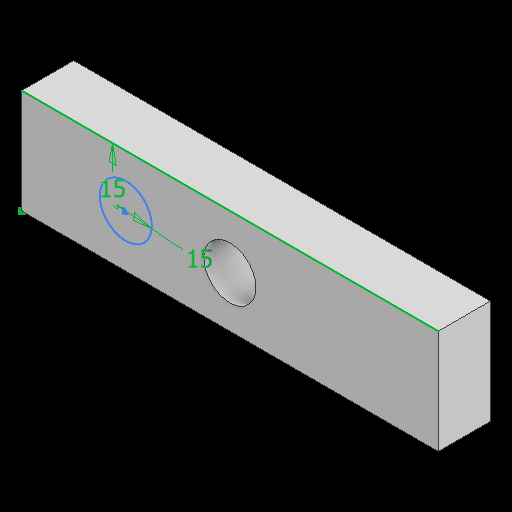
# Autodesk Inventor part: lever1.2
Saved by Autodesk Inventor 2025.1 (Build 291241000, 241)
## iProperties
Created: 2024-08-22
Part Number: lever1.2
Material: 일반
Document SubType Name: Modeling
Designer: ojs08
Density: 1 g/cm^3
Appearance: 기본값
Author: ojs08
Autodesk Inventor part; units mm, degrees
ref_plane "YZ Plane" through (0, 0, 0) normal (1, 0, 0) x (0, 1, 0)
ref_plane "XZ Plane" through (0, 0, 0) normal (0, 1, 0) x (-1, 0, 0)
ref_plane "XY Plane" through (0, 0, 0) normal (0, 0, 1) x (1, 0, 0)
sketch "스케치1" plane through (0, 0, 0) normal (0, 0, 1) x (1, 0, 0)
  line L0 (0, 30) -> (120, 30)
  line L1 (120, 30) -> (120, 0)
  line L2 (120, 0) -> (0, 0)
  line L3 (0, 0) -> (0, 30)
  dimension "d0" = 120
  dimension "d1" = 30
  constraints: 8 end point, 2 parallel, 1 coincident, 1 horizontal, 1 perpendicular
  measures "d0" distance of L0.start L0.end
  measures "d1" distance of L2.end L0.start
extrude "돌출1" add sketch "스케치1" along normal blind 15
sketch "스케치2" plane through (0, 0, 15) normal (0, 0, 1) x (1, 0, 0)
  circle A0 centre (30, 15) radius 7.5
  line L0 (120, 30) -> (0, 30) projected
  point P0 (0, 0)
  dimension "d4" = 15
  dimension "d5" = 15
  constraints: 1 centre point
  measures "d4" diameter of A0
  measures "d5" distance from line of L0 A0.centre
sketch "스케치3" plane through (0, 0, 15) normal (0, 0, 1) x (1, 0, 0)
  circle A0 centre (60, 14.5644) radius 7.5
  line L0 (0, 30) -> (0, 0) projected
  dimension "d8" = 60
  constraints: 1 centre point
  measures "d8" distance from line of L0 A0.centre
extrude "돌출2" cut sketch "스케치3" against normal up to surface (15 mm away)
